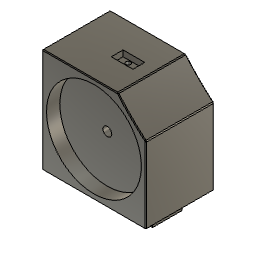
Laser Pulse Holder (Autodesk Fusion 360 design; units mm, degrees)
Autodesk Fusion 360 part; units mm, degrees
sketch "Sketch1" plane through (0, 0, 0) normal (0, 0, 1) x (1, 0, 0)
  line L0 (13.25, 5) -> (-13.25, 5)
  line L1 (-13.25, 5) -> (-13.25, -5)
  line L2 (-13.25, -5) -> (13.25, -5)
  line L3 (13.25, -5) -> (13.25, 5)
  line L4 (13.25, 5) -> (-13.25, -5) construction
  line L5 (-13.25, 5) -> (13.25, -5) construction
  line L6 (2.65, -1) -> (-2.65, -1)
  line L7 (-2.65, -1) -> (-2.65, 1)
  line L8 (-2.65, 1) -> (2.65, 1)
  line L9 (2.65, 1) -> (2.65, -1)
  line L10 (2.65, -1) -> (-2.65, 1) construction
  line L11 (-2.65, -1) -> (2.65, 1) construction
  dimension "d1" = 26.5
  dimension "d2" = 10
  dimension "d3" = 5.3
  dimension "d4" = 2
  constraint horizontal L0
  constraint perpendicular L0 L1
  constraint parallel L0 L2
  constraint parallel L1 L3
  constraint coincident L4 origin
  constraint coincident L5 origin
  constraint horizontal L6
  constraint perpendicular L6 L7
  constraint parallel L6 L8
  constraint parallel L7 L9
  constraint coincident L10 origin
  constraint coincident L11 origin
  measures "d1" distance of L1.end L2.end
  measures "d2" distance of L0.end L1.end
  measures "d3" distance of L7.end L8.end
  measures "d4" distance of L6.end L7.end
extrude "Extrude1" add sketch "Sketch1" along normal blind 5 makes body 1
sketch "Sketch2" plane through (0, 0, 5) normal (0, 0, 1) x (-1, 0, 0)
  line L0 (2.65, -1) -> (-2.65, -1)
  line L1 (-2.65, -1) -> (-2.65, 1)
  line L2 (-2.65, 1) -> (2.65, 1)
  line L3 (2.65, 1) -> (2.65, -1)
  line L4 (-13.25, 5) -> (-13.25, -5)
  line L5 (-13.25, -5) -> (13.25, -5)
  line L6 (13.25, -5) -> (13.25, 5)
  line L7 (13.25, 5) -> (-13.25, 5)
  line L8 (-17.5, -17.5) -> (17.5, -17.5)
  line L9 (17.5, -17.5) -> (17.5, 17.5)
  line L10 (17.5, 17.5) -> (-17.5, 17.5)
  line L11 (-17.5, 17.5) -> (-17.5, -17.5)
  line L12 (-17.5, -17.5) -> (17.5, 17.5) construction
  line L13 (17.5, -17.5) -> (-17.5, 17.5) construction
  line L14 (-2.65, -1) -> (2.65, -1)
  line L15 (2.65, -1) -> (2.65, 1)
  line L16 (2.65, 1) -> (-2.65, 1)
  line L17 (-2.65, 1) -> (-2.65, -1)
  line L18 (-2.65, -1) -> (2.65, 1) construction
  line L19 (2.65, -1) -> (-2.65, 1) construction
  dimension "d7" = 35
  dimension "d8" = 35
  constraint horizontal L8
  constraint perpendicular L8 L9
  constraint parallel L8 L10
  constraint parallel L9 L11
  constraint coincident L12 origin
  constraint coincident L13 origin
  constraint horizontal L14
  constraint perpendicular L14 L15
  constraint parallel L14 L16
  constraint parallel L15 L17
  constraint coincident L0.end L1.start
  constraint coincident L18 origin
  constraint coincident L19 origin
  measures "d7" distance of L9.end L10.end
  measures "d8" distance of L8.end L9.end
extrude "Extrude2" add sketch "Sketch2" along normal blind 35 contours L4 L5 L6 L7 | L8 L9 L10 L11 bodies 1
chamfer "Chamfer1" distance 3.5 angle 45 2 edges at (0, -1, 0) (0, 1, 0) on bodies 1
chamfer "Chamfer2" distance 10.1 angle 45 2 edges at (2.65, 0, 0) (-2.65, 0, 0) on bodies 1
extrude "Extrude3" cut 1 faces at (5.8333, -17.5, 28.3333) along direction (0, 1, 0) blind 6 on bodies 1 bodies 1
extrude "Extrude4" cut 1 faces at (-5.8333, 17.5, 28.3333) along direction (0, -1, 0) blind 6 on bodies 1 bodies 1
sketch "Sketch3" plane through (0, -11.5, 0) normal (0, -1, 0) x (1, 0, 0)
  line L0 (-17.5, 5) -> (17.5, 5)
  line L1 (17.5, 5) -> (17.5, 40)
  line L2 (17.5, 40) -> (-17.5, 40)
  line L3 (-17.5, 40) -> (-17.5, 5)
  line L4 (0, 40) -> (0, 22.5)
  circle A0 centre (0, 22.5) radius 17
  dimension "d17" = 17.5
  dimension "d18" = 34
  constraint midpoint L2 L4.start
  constraint perpendicular L0 L4
  constraint coincident L4.end A0.centre
  measures "d17" distance of L4.start L4.end
  measures "d18" diameter of A0
extrude "Extrude5" cut sketch "Sketch3" against normal blind 4.5 contours A0 bodies 1
sketch "Sketch4" plane through (0, -7, 0) normal (0, -1, 0) x (1, 0, 0)
  circle A0 centre (0, 22.5) radius 17
  circle A1 centre (0, 22.5) radius 1.5
  dimension "d21" = 3
  constraint concentric A0 A1
  measures "d21" diameter of A1
extrude "Extrude6" cut sketch "Sketch4" against normal blind 6 contours A1 bodies 1
sketch "Sketch5" plane through (0, 11.5, 0) normal (0, 1, 0) x (-1, 0, 0)
  line L0 (-17.5, 5) -> (17.5, 5)
  line L1 (17.5, 5) -> (17.5, 40)
  line L2 (17.5, 40) -> (-17.5, 40)
  line L3 (-17.5, 40) -> (-17.5, 5)
  line L4 (0, 40) -> (0, 22.5)
  line L5 (0, 22.5) -> (-70.7107, 93.2107)
  line L6 (0, 22.5) -> (100, 22.5) construction
  circle A0 centre (-70.7107, 93.2107) radius 82.2239
  dimension "d24" = 17.5
  dimension "d25" = 135
  dimension "d26" = 100
  constraint midpoint L2 L4.start
  constraint perpendicular L2 L4
  constraint horizontal L6
  constraint coincident L5.end A0.centre
  measures "d24" distance of L4.start L4.end
  measures "d25" angle of L5 L6
  measures "d26" distance of L4.end L5.end
extrude "Extrude7" cut sketch "Sketch5" against normal blind 25 contours L3 L5 A0 | L2 L5 A0 bodies 1
chamfer "Chamfer3" distance 1 angle 45 4 edges at (0, 1, 40) (-2.65, 0, 40) (2.65, 0, 40) (0, -1, 40) on bodies 1
chamfer "Chamfer4" distance 0.25 angle 45 11 edges at (8.0258, 0, 40) (17.5, 0, 30.5258) (12.5696, -11.5, 35.0696) (-4.7371, -11.5, 40) (-4.7371, 11.5, 40) (12.5696, 11.5, 35.0696) (17.5, 11.5, 17.7629) (17.5, -11.5, 17.7629) (-17.5, -11.5, 22.5) (-17.5, 0, 40) (-17.5, 11.5, 22.5) on bodies 1
move_face "OffsetFaces1" offset 1 1 faces at (16.9789, -10, 23.3474) on bodies 1
sketch "Sketch6" plane through (0, 0, 0) normal (0, 0, 1) x (1, 0, 0)
  circle A0 centre (42.0682, -1.7821) radius 0.8
  circle A1 centre (42.0682, -1.7821) radius 1.3459
  dimension "d32" = 1.6
  dimension "d33" = 0.5459
  measures "d32" diameter of A0
extrude "Extrude8" add sketch "Sketch6" along normal blind 20 separate body makes body 2
move_body "Move1" bodies 2 to x (1, 0, 0) y (0, 1, 0) z (0, 0, 1) at (-42, 2, 0)
move_body "Move2" bodies 2 to x (1, 0, 0) y (0, 1, 0) z (0, 0, 1) at (0, -0.2, 0)
extrude "Extrude9" cut 1 faces at (1.2271, -0.0489, 0) along direction (0, 0, 1) blind 3 on bodies 2 bodies 2
extrude "Extrude10" add 1 faces at (-2.65, 0.3333, 19.7333) along direction (1, 0, 0) blind 1.85 on bodies 1 bodies 1 2
extrude "Extrude11" cut 1 faces at (2.65, -0.3333, 19.7333) along direction (-1, 0, 0) blind 1.4 on bodies 1 bodies 1
extrude "Extrude12" cut 1 faces at (2.65, -0.3333, 19.7333) along direction (-1, 0, 0) blind 1.65 on bodies 1 bodies 1
extrude "Extrude13" add 1 faces at (0.0922, -0.9266, 20) along direction (0, 0, 1) blind 19 on bodies 1 bodies 1
delete_face "DeleteFace1" 1 faces at (1.1757, 0.7826, 5.3667) on bodies 1
extrude "Extrude14" add 1 faces at (-2.0106, 0.006, 10.1) along direction (0, 0, -1) blind 6.57 on bodies 1 bodies 1
extrude "Extrude15" cut 1 faces at (1, 0.3333, 21.304) along direction (1, 0, 0) blind 2 on bodies 1 bodies 1
extrude "Extrude16" add 1 faces at (1, 0.3333, 21.304) along direction (1, 0, 0) blind 2 on bodies 1 bodies 1
extrude "Extrude17" cut 1 faces at (-0.1387, -1, 22.2597) along direction (0, 1, 0) blind 1 on bodies 1 bodies 1
extrude "Extrude18" cut 1 faces at (3, 0.3333, 5.6033) along direction (1, 0, 0) blind 6 on bodies 1 bodies 1
